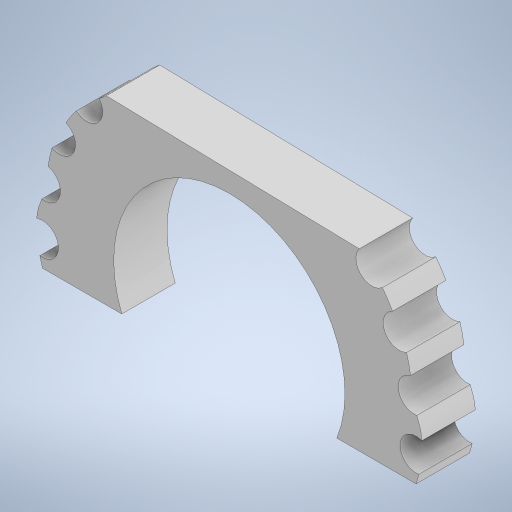
# Autodesk Inventor part: бок пуска держатель диодов
Saved by Autodesk Inventor 2023.1 (Build 271208000, 208)
## iProperties
Created: 2023-04-05
Part Number: бок пуска держатель диодов
Material: Типовые
Document SubType Name: Modeling
Designer: User
Density: 1 g/cm^3
Appearance: По умолчанию
Author: User
Autodesk Inventor part; units mm, degrees
(part 1 of 4)
ref_plane "YZ Plane" through (0, 0, 0) normal (1, 0, 0) x (0, 1, 0)
ref_plane "XZ Plane" through (0, 0, 0) normal (0, 1, 0) x (-1, 0, 0)
ref_plane "XY Plane" through (0, 0, 0) normal (0, 0, 1) x (1, 0, 0)
sketch "Эскиз1" plane through (0, 0, 0) normal (0, 0, 1) x (1, 0, 0)
  line L0 (-15.4323, 26.5556) -> (-15.4323, 37)
  line L1 (-15.4323, 37) -> (-36, 37)
  line L2 (-36, 37) -> (-36, 61)
  line L3 (-36, 61) -> (35, 61)
  line L4 (35, 61) -> (35, 37)
  line L5 (35, 37) -> (15.4323, 37)
  line L6 (15.4323, 37) -> (15.4323, 26.5556)
  line L7 (15.4323, 26.5556) -> (13.136, 23.9434)
  line L8 (11.832, 23.9746) -> (14.4323, 26.9326)
  line L9 (14.4323, 26.9326) -> (14.4323, 37)
  line L10 (14.4323, 37) -> (-14.4323, 37)
  line L11 (-14.4323, 37) -> (-14.4323, 26.9326)
  line L12 (-14.4323, 26.9326) -> (-12.3404, 24.5529)
  line L13 (-13.7005, 24.5855) -> (-15.4323, 26.5556)
  line L14 (39, 3.2152) -> (19.5419, 3.2152)
  line L15 (19.5419, 3.2152) -> (16.1608, 4.2152)
  line L16 (19.6867, 4.2152) -> (39, 4.2152)
  line L17 (39, 4.2152) -> (39, 63.4697)
  arc A0 (39, 63.4697) -> (38, 64.4697) centre (38, 63.4697) ccw
  line L18 (38, 64.4697) -> (10.2401, 64.4697)
  line L19 (10.2401, 64.4697) -> (10.2401, 65.4697)
  line L20 (10.2401, 65.4697) -> (38, 65.4697)
  arc A1 (40, 63.4697) -> (38, 65.4697) centre (38, 63.4697) ccw
  line L21 (40, 63.4697) -> (40, -99.0936)
  arc A2 (33, -106.0936) -> (40, -99.0936) centre (33, -99.0936) ccw
  line L22 (33, -106.0936) -> (-33, -106.0936)
  arc A3 (-40, -99.0936) -> (-33, -106.0936) centre (-33, -99.0936) ccw
  line L23 (-40, -99.0936) -> (-40, 63.4697)
  arc A4 (-38, 65.4697) -> (-40, 63.4697) centre (-38, 63.4697) ccw
  line L24 (-38, 65.4697) -> (-10.1221, 65.4697)
  line L25 (-10.1221, 65.4697) -> (-10.1221, 64.4697)
  line L26 (-10.1221, 64.4697) -> (-38, 64.4697)
  arc A5 (-38, 64.4697) -> (-39, 63.4697) centre (-38, 63.4697) ccw
  line L27 (-39, 63.4697) -> (-39, 4.2152)
  line L28 (-39, 4.2152) -> (-19.6867, 4.2152)
  line L29 (-16.1608, 4.2152) -> (-19.5419, 3.2152)
  line L30 (-19.5419, 3.2152) -> (-39, 3.2152)
  line L31 (-39, 3.2152) -> (-39, -99.0936)
  arc A6 (-39, -99.0936) -> (-33, -105.0936) centre (-33, -99.0936) ccw
  line L32 (-33, -105.0936) -> (33, -105.0936)
  arc A7 (33, -105.0936) -> (39, -99.0936) centre (33, -99.0936) ccw
  line L33 (39, -99.0936) -> (39, 3.2152)
  line L34 (34.3097, 25.5954) -> (34.3097, 24.7932)
  line L35 (34.3097, 24.7932) -> (34.257, 24.7932)
  line L36 (34.2611, 22.0622) -> (34.3097, 22.0622)
  line L37 (34.3097, 22.0622) -> (34.3097, 21.268)
  line L38 (27.8227, 25.9277) -> (28.6411, 25.9277)
  line L39 (28.6411, 25.9277) -> (30.3267, 20.9277)
  line L40 (30.3267, 20.9277) -> (29.6257, 20.9277)
  line L41 (29.6257, 20.9277) -> (29.1719, 22.3256)
  line L42 (29.1719, 22.3256) -> (27.2635, 22.3256)
  line L43 (27.2635, 22.3256) -> (26.8097, 20.9277)
  line L44 (26.8097, 20.9277) -> (26.1371, 20.9277)
  line L45 (26.1371, 20.9277) -> (27.8227, 25.9277)
  line L46 (24.0706, 20.9277) -> (22.6241, 20.9277)
  line L47 (22.6241, 20.9277) -> (22.6241, 25.9277)
  line L48 (22.6241, 25.9277) -> (25.6671, 25.9277)
  line L49 (25.6671, 25.9277) -> (25.6671, 25.3361)
  line L50 (25.6671, 25.3361) -> (23.2886, 25.3361)
  line L51 (23.2886, 25.3361) -> (23.2886, 23.9666)
  line L52 (23.2886, 23.9666) -> (24.0909, 23.9666)
  line L53 (26.6314, 29.3789) -> (26.6314, 30.0758)
  line L54 (26.6314, 30.0758) -> (26.6719, 30.0758)
  line L55 (27.8956, 30.8456) -> (27.4539, 30.8456)
  line L56 (27.4539, 30.8456) -> (27.4539, 31.3886)
  line L57 (27.4539, 31.3886) -> (27.7943, 31.3886)
  line L58 (26.8543, 32.1098) -> (26.8138, 32.1098)
  line L59 (26.8138, 32.1098) -> (26.8138, 32.7905)
  line L60 (24.7149, 32.9121) -> (26.0642, 32.9121)
  line L61 (26.0642, 32.9121) -> (26.0642, 29.1601)
  line L62 (26.0642, 29.1601) -> (25.4321, 29.1601)
  line L63 (25.4321, 29.1601) -> (25.4321, 30.6471)
  line L64 (25.4321, 30.6471) -> (24.8121, 30.6471)
  line L65 (24.8121, 30.6471) -> (23.6979, 29.1601)
  line L66 (23.6979, 29.1601) -> (22.9604, 29.1601)
  line L67 (22.9604, 29.1601) -> (24.1679, 30.7038)
  line L68 (19.1679, 32.7095) -> (19.1679, 32.0004)
  line L69 (19.1679, 32.0004) -> (19.1314, 32.0004)
  line L70 (19.1314, 30.0798) -> (19.1679, 30.0798)
  line L71 (19.1679, 30.0798) -> (19.1679, 29.3707)
  line L72 (-26.95, 20.6933) -> (-28.3965, 20.6933)
  line L73 (-28.3965, 20.6933) -> (-28.3965, 25.6933)
  line L74 (-28.3965, 25.6933) -> (-25.3535, 25.6933)
  line L75 (-25.3535, 25.6933) -> (-25.3535, 25.1017)
  line L76 (-25.3535, 25.1017) -> (-27.732, 25.1017)
  line L77 (-27.732, 25.1017) -> (-27.732, 23.7322)
  line L78 (-27.732, 23.7322) -> (-26.9297, 23.7322)
  line L79 (-37.0634, 29.1444) -> (-37.0634, 29.8414)
  line L80 (-37.0634, 29.8414) -> (-37.0229, 29.8414)
  line L81 (-35.7992, 30.6112) -> (-36.2409, 30.6112)
  line L82 (-36.2409, 30.6112) -> (-36.2409, 31.1542)
  line L83 (-36.2409, 31.1542) -> (-35.9005, 31.1542)
  line L84 (-36.8406, 31.8754) -> (-36.8811, 31.8754)
  line L85 (-36.8811, 31.8754) -> (-36.8811, 32.5561)
  line L86 (-33.4978, 31.9524) -> (-33.5342, 31.9524)
  line L87 (-33.5342, 31.9524) -> (-33.5342, 32.5966)
  line L88 (-30.8479, 31.4905) -> (-30.8479, 28.9256)
  line L89 (-30.8479, 28.9256) -> (-31.4799, 28.9256)
  line L90 (-31.4799, 28.9256) -> (-31.4799, 29.3227)
  line L91 (-29.3284, 29.1161) -> (-29.3284, 27.544)
  line L92 (-29.3284, 27.544) -> (-29.9605, 27.544)
  line L93 (-29.9605, 27.544) -> (-29.9605, 32.6777)
  line L94 (-29.9605, 32.6777) -> (-29.3284, 32.6777)
  line L95 (-29.3284, 32.6777) -> (-29.3284, 32.2846)
  line L96 (-24.7944, 32.6777) -> (-23.4451, 32.6777)
  line L97 (-23.4451, 32.6777) -> (-23.4451, 28.9256)
  line L98 (-23.4451, 28.9256) -> (-24.0772, 28.9256)
  line L99 (-24.0772, 28.9256) -> (-24.0772, 30.4127)
  line L100 (-24.0772, 30.4127) -> (-24.6971, 30.4127)
  line L101 (-24.6971, 30.4127) -> (-25.8114, 28.9256)
  line L102 (-25.8114, 28.9256) -> (-26.5488, 28.9256)
  line L103 (-26.5488, 28.9256) -> (-25.3414, 30.4694)
  line L104 (-21.9864, 32.6777) -> (-19.689, 32.6777)
  line L105 (-19.689, 32.6777) -> (-19.689, 29.4645)
  line L106 (-19.689, 29.4645) -> (-19.3162, 29.4645)
  line L107 (-19.3162, 29.4645) -> (-19.3162, 28.0261)
  line L108 (-19.3162, 28.0261) -> (-19.9038, 28.0261)
  line L109 (-19.9038, 28.0261) -> (-19.9038, 28.9337)
  line L110 (-19.9038, 28.9337) -> (-22.3714, 28.9337)
  line L111 (-22.3714, 28.9337) -> (-22.3714, 28.0261)
  line L112 (-22.3714, 28.0261) -> (-22.9589, 28.0261)
  line L113 (-22.9589, 28.0261) -> (-22.9589, 29.4645)
  line L114 (-22.9589, 29.4645) -> (-22.7117, 29.4645)
  line L115 (-35.5196, 25.6933) -> (-34.7012, 25.6933)
  line L116 (-34.7012, 25.6933) -> (-33.0156, 20.6933)
  line L117 (-33.0156, 20.6933) -> (-33.7166, 20.6933)
  line L118 (-33.7166, 20.6933) -> (-34.1704, 22.0912)
  line L119 (-34.1704, 22.0912) -> (-36.0788, 22.0912)
  line L120 (-36.0788, 22.0912) -> (-36.5326, 20.6933)
  line L121 (-36.5326, 20.6933) -> (-37.2052, 20.6933)
  line L122 (-37.2052, 20.6933) -> (-35.5196, 25.6933)
  line L123 (-30.8722, 23.3229) -> (-28.8422, 20.6933)
  line L124 (-28.8422, 20.6933) -> (-29.689, 20.6933)
  line L125 (-29.689, 20.6933) -> (-31.4597, 22.9866)
  line L126 (-31.4597, 22.9866) -> (-31.877, 22.9866)
  line L127 (-31.877, 22.9866) -> (-31.877, 20.6933)
  line L128 (-31.877, 20.6933) -> (-32.5415, 20.6933)
  line L129 (-32.5415, 20.6933) -> (-32.5415, 25.6933)
  line L130 (-32.5415, 25.6933) -> (-31.877, 25.6933)
  line L131 (-31.877, 25.6933) -> (-31.877, 23.4404)
  line L132 (-29.3122, 25.6933) -> (-29.1055, 25.6933)
  line L133 (-29.1055, 25.6933) -> (-29.1055, 25.1017)
  line L134 (-29.1055, 25.1017) -> (-29.2717, 25.1017)
  line L135 (21.2181, 29.1601) -> (19.7432, 29.1601)
  line L136 (19.7432, 29.1601) -> (19.7432, 32.9121)
  line L137 (19.7432, 32.9121) -> (21.1209, 32.9121)
  line L138 (31.4369, 29.1601) -> (30.1241, 29.1601)
  line L139 (30.1241, 29.1601) -> (30.1241, 32.9121)
  line L140 (30.1241, 32.9121) -> (30.7562, 32.9121)
  line L141 (30.7562, 32.9121) -> (30.7562, 31.4494)
  line L142 (30.7562, 31.4494) -> (31.4531, 31.4494)
  line L143 (38.3089, 32.7095) -> (38.3089, 32.0004)
  line L144 (38.3089, 32.0004) -> (38.2724, 32.0004)
  line L145 (38.2724, 30.0798) -> (38.3089, 30.0798)
  line L146 (38.3089, 30.0798) -> (38.3089, 29.3707)
  line L147 (36.0601, 21.9609) -> (36.1776, 22.2243)
  line L148 (36.1776, 22.2243) -> (34.4191, 25.9277)
  line L149 (34.4191, 25.9277) -> (35.1565, 25.9277)
  line L150 (35.1565, 25.9277) -> (36.5139, 22.986)
  line L151 (36.5139, 22.986) -> (37.7376, 25.9277)
  line L152 (37.7376, 25.9277) -> (38.4223, 25.9277)
  line L153 (38.4223, 25.9277) -> (36.6071, 21.7178)
  line L154 (34.9013, 20.9277) -> (34.9013, 21.5517)
  line L155 (34.9013, 21.5517) -> (34.9499, 21.5517)
  line L156 (-5.6509, -41.2421) -> (-5.6509, -36.154)
  line L157 (-5.6509, -36.154) -> (-8.0452, -36.154)
  line L158 (-8.0452, -36.154) -> (-8.0452, -41.2421)
  line L159 (-34.9687, -1.889) -> (-34.9687, -0.3964)
  line L160 (-34.9687, -0.3964) -> (-36.2158, -0.3964)
  line L161 (-36.2158, 0.1024) -> (-34.9687, 0.1024)
  line L162 (-34.9687, 0.1024) -> (-34.9687, 1.104)
  line L163 (-26.4317, -100.2362) -> (-26.4317, -101.232)
  line L164 (-26.4317, -101.232) -> (-26.032, -101.232)
  line L165 (-28.4267, -102.8274) -> (-29.2227, -102.8274)
  line L166 (-29.2227, -102.8274) -> (-29.2227, -103.8232)
  line L167 (5.095, 27.3433) -> (4.0974, 28.8866)
  line L168 (4.0974, 28.8866) -> (3.5401, 28.302)
  line L169 (3.5401, 28.302) -> (3.5401, 27.5031)
  line L170 (3.5401, 30.4961) -> (3.5401, 29.023)
  line L171 (3.5401, 29.023) -> (5.1223, 30.6831)
  line L172 (5.4497, 30.3051) -> (4.4481, 29.249)
  line L173 (4.4481, 29.249) -> (5.473, 27.6629)
  line L174 (-1.3976, 26.7549) -> (-1.3976, 27.2537)
  line L175 (-1.3976, 27.2537) -> (-2.3952, 27.2537)
  line L176 (-2.3952, 27.7525) -> (-1.3976, 27.7525)
  line L177 (-1.3976, 27.7525) -> (-1.3976, 30.4961)
  line L178 (6.3343, 34.5821) -> (6.3343, 33.335)
  line L179 (6.3343, 33.335) -> (7.8308, 33.335)
  line L180 (7.8308, 33.335) -> (7.8308, 34.5821)
  line L181 (7.8308, 31.5891) -> (7.8308, 32.8362)
  line L182 (7.8308, 32.8362) -> (6.3343, 32.8362)
  line L183 (6.3343, 32.8362) -> (6.3343, 31.5891)
  line L184 (4.5884, 32.8362) -> (2.8425, 32.8362)
  line L185 (2.8425, 32.8362) -> (2.8425, 32.3374)
  line L186 (-4.64, 31.5891) -> (-4.64, 34.3327)
  line L187 (-4.64, 34.3327) -> (-5.6376, 34.3327)
  line L188 (-5.6376, 34.3327) -> (-5.6376, 31.5891)
  line L189 (-3.6423, 34.3327) -> (-4.1411, 34.3327)
  line L190 (-4.1411, 34.3327) -> (-4.1411, 31.5891)
  line L191 (0.3136, 63.3342) -> (0.3136, 66.0778)
  line L192 (0.3136, 66.0778) -> (-0.2592, 66.0778)
  line L193 (-0.2592, 66.0778) -> (-1.1945, 63.2563)
  line L194 (-1.6778, 63.3225) -> (-1.6622, 63.4122)
  line L195 (-1.6622, 63.4122) -> (-0.6723, 66.4052)
  line L196 (-7.1688, 66.0778) -> (-8.1665, 66.0778)
  line L197 (-8.1665, 66.0778) -> (-8.1665, 63.3342)
  line L198 (4.0549, 64.5813) -> (2.309, 64.5813)
  line L199 (2.309, 64.5813) -> (2.309, 64.0825)
  line L200 (6.7984, 63.3342) -> (6.7984, 66.0778)
  line L201 (6.7984, 66.0778) -> (5.8008, 66.0778)
  line L202 (5.8008, 66.0778) -> (5.8008, 63.3342)
  line L203 (7.7961, 66.0778) -> (7.2973, 66.0778)
  line L204 (7.2973, 66.0778) -> (7.2973, 63.3342)
  line L205 (0.8472, 31.5891) -> (0.8472, 33.8066)
  line L206 (0.8472, 33.8066) -> (0.0521, 32.692)
  line L207 (-0.3532, 32.692) -> (-1.1482, 33.8066)
  line L208 (-1.1482, 33.8066) -> (-1.1482, 31.5891)
  line L209 (-1.1949, 34.7263) -> (-0.1505, 33.2649)
  line L210 (-0.1505, 33.2649) -> (0.8939, 34.7263)
  line L211 (-5.3882, 30.2467) -> (-6.3859, 30.2467)
  line L212 (-6.3859, 30.2467) -> (-6.3859, 27.5031)
  line L213 (-32.017, -102.6276) -> (-32.017, -100.436)
  line L214 (-32.017, -100.436) -> (-32.813, -100.436)
  line L215 (-32.813, -100.436) -> (-32.813, -102.6276)
  line L216 (-31.2177, -100.436) -> (-31.6174, -100.436)
  line L217 (-31.6174, -100.436) -> (-31.6174, -102.6276)
  line L218 (-23.9945, -2.6373) -> (-23.9945, 1.6028)
  line L219 (-23.9945, 1.6028) -> (-25.9898, 1.6028)
  line L220 (-25.9898, 1.6028) -> (-25.9898, -2.6373)
  line L221 (-0.8621, -40.3442) -> (-0.8621, -39.147)
  line L222 (-0.8621, -39.147) -> (-2.6579, -39.147)
  line L223 (-2.6579, -38.5484) -> (-0.8621, -38.5484)
  line L224 (-0.8621, -38.5484) -> (-0.8621, -35.8547)
  line L225 (5.7225, -35.8454) -> (5.7225, -38.1369)
  line L226 (5.7225, -38.1369) -> (8.2385, -35.6349)
  line L227 (8.6594, -36.0652) -> (6.8776, -37.8423)
  line L228 (6.8776, -37.8423) -> (8.7155, -41.0924)
  line L229 (8.7155, -41.0924) -> (8.7576, -41.2514)
  line L230 (8.187, -41.3824) -> (6.438, -38.2631)
  line L231 (6.438, -38.2631) -> (5.7225, -38.9646)
  line L232 (5.7225, -38.9646) -> (5.7225, -41.2421)
  line L233 (26.4641, 0.963) -> (26.659, 0.963)
  line L234 (26.659, 0.963) -> (25.5405, 2.027)
  line L235 (27.7112, 1.9607) -> (26.3394, 1.9607)
  line L236 (26.3394, 1.9607) -> (27.6605, 0.698)
  line L237 (27.6605, 0.698) -> (27.7229, 0.6162)
  line L238 (30.4548, -2.5288) -> (29.4571, -2.5288)
  line L239 (29.4571, -2.5288) -> (29.4571, -3.7758)
  arc A8 (-45, -109) -> (-42, -112) centre (-42, -109) ccw
  line L240 (-42, -112) -> (42, -112)
  arc A9 (42, -112) -> (45, -109) centre (42, -109) ccw
  line L241 (45, -109) -> (45, 108)
  arc A10 (45, 108) -> (42, 111) centre (42, 108) ccw
  line L242 (42, 111) -> (-42, 111)
  arc A11 (-42, 111) -> (-45, 108) centre (-42, 108) ccw
  line L243 (-45, 108) -> (-45, -109)
  line L244 (-30.3205, -53.3887) -> (-30.3205, -51.1972)
  line L245 (-30.3205, -51.1972) -> (-31.1165, -51.1972)
  line L246 (-31.1165, -51.1972) -> (-31.1165, -53.3887)
  line L247 (-29.5212, -51.1972) -> (-29.9208, -51.1972)
  line L248 (-29.9208, -51.1972) -> (-29.9208, -53.3887)
  arc A12 (37, 68) -> (40, 71) centre (37, 71) ccw
  line L249 (37, 68) -> (-37, 68)
  arc A13 (-40, 71) -> (-37, 68) centre (-37, 71) ccw
  line L250 (-40, 71) -> (-40, 102)
  arc A14 (-33, 109) -> (-40, 102) centre (-33, 102) ccw
  line L251 (-33, 109) -> (33, 109)
  arc A15 (40, 102) -> (33, 109) centre (33, 102) ccw
  line L252 (40, 102) -> (40, 71)
  circle A16 centre (-32, -94) radius 5
  circle A17 centre (-32, -44.7228) radius 5
  spline S0 degree 2 poles (31.1452, 21.4949) (30.8454, 21.8191) (30.5172, 22.7915) (30.5172, 23.4236) knots 0 0 0 1 2 2 2
  line L253 (31.1452, 21.4949) -> (30.8454, 21.8191) construction
  line L254 (30.8454, 21.8191) -> (30.5172, 22.7915) construction
  line L255 (30.5172, 22.7915) -> (30.5172, 23.4236) construction
  spline S1 degree 2 poles (30.5172, 23.4236) (30.5172, 24.0517) (30.8373, 24.9836) (31.1411, 25.328) knots 0 0 0 1 2 2 2
  line L256 (30.5172, 23.4236) -> (30.5172, 24.0517) construction
  line L257 (30.5172, 24.0517) -> (30.8373, 24.9836) construction
  line L258 (30.8373, 24.9836) -> (31.1411, 25.328) construction
  spline S2 degree 2 poles (31.1411, 25.328) (31.441, 25.6643) (32.2595, 26.0168) (32.7659, 26.0168) knots 0 0 0 1 2 2 2
  line L259 (31.1411, 25.328) -> (31.441, 25.6643) construction
  line L260 (31.441, 25.6643) -> (32.2595, 26.0168) construction
  line L261 (32.2595, 26.0168) -> (32.7659, 26.0168) construction
  spline S3 degree 2 poles (32.7659, 26.0168) (33.0172, 26.0168) (33.4588, 25.9439) (33.6452, 25.8872) knots 0 0 0 1 2 2 2
  line L262 (32.7659, 26.0168) -> (33.0172, 26.0168) construction
  line L263 (33.0172, 26.0168) -> (33.4588, 25.9439) construction
  line L264 (33.4588, 25.9439) -> (33.6452, 25.8872) construction
  spline S4 degree 2 poles (33.6452, 25.8872) (33.8073, 25.8345) (34.1436, 25.6846) (34.3097, 25.5954) knots 0 0 0 1 2 2 2
  line L265 (33.6452, 25.8872) -> (33.8073, 25.8345) construction
  line L266 (33.8073, 25.8345) -> (34.1436, 25.6846) construction
  line L267 (34.1436, 25.6846) -> (34.3097, 25.5954) construction
  spline S5 degree 2 poles (34.257, 24.7932) (34.1679, 24.8742) (33.8924, 25.1011) (33.6938, 25.2105) knots 0 0 0 1 2 2 2
  line L268 (34.257, 24.7932) -> (34.1679, 24.8742) construction
  line L269 (34.1679, 24.8742) -> (33.8924, 25.1011) construction
  line L270 (33.8924, 25.1011) -> (33.6938, 25.2105) construction
  spline S6 degree 2 poles (33.6938, 25.2105) (33.5034, 25.3159) (33.0536, 25.4496) (32.7619, 25.4496) knots 0 0 0 1 2 2 2
  line L271 (33.6938, 25.2105) -> (33.5034, 25.3159) construction
  line L272 (33.5034, 25.3159) -> (33.0536, 25.4496) construction
  line L273 (33.0536, 25.4496) -> (32.7619, 25.4496) construction
  spline S7 degree 2 poles (32.7619, 25.4496) (32.4418, 25.4496) (31.8705, 25.1862) (31.6557, 24.935) knots 0 0 0 1 2 2 2
  line L274 (32.7619, 25.4496) -> (32.4418, 25.4496) construction
  line L275 (32.4418, 25.4496) -> (31.8705, 25.1862) construction
  line L276 (31.8705, 25.1862) -> (31.6557, 24.935) construction
  spline S8 degree 2 poles (31.6557, 24.935) (31.445, 24.6797) (31.21, 23.9058) (31.21, 23.4236) knots 0 0 0 1 2 2 2
  line L277 (31.6557, 24.935) -> (31.445, 24.6797) construction
  line L278 (31.445, 24.6797) -> (31.21, 23.9058) construction
  line L279 (31.21, 23.9058) -> (31.21, 23.4236) construction
  spline S9 degree 2 poles (31.21, 23.4236) (31.21, 22.909) (31.4572, 22.1676) (31.6719, 21.9123) knots 0 0 0 1 2 2 2
  line L280 (31.21, 23.4236) -> (31.21, 22.909) construction
  line L281 (31.21, 22.909) -> (31.4572, 22.1676) construction
  line L282 (31.4572, 22.1676) -> (31.6719, 21.9123) construction
  spline S10 degree 2 poles (31.6719, 21.9123) (31.8826, 21.6651) (32.4458, 21.4139) (32.7619, 21.4139) knots 0 0 0 1 2 2 2
  line L283 (31.6719, 21.9123) -> (31.8826, 21.6651) construction
  line L284 (31.8826, 21.6651) -> (32.4458, 21.4139) construction
  line L285 (32.4458, 21.4139) -> (32.7619, 21.4139) construction
  spline S11 degree 2 poles (32.7619, 21.4139) (33.0496, 21.4139) (33.5398, 21.5557) (33.7303, 21.6611) knots 0 0 0 1 2 2 2
  line L286 (32.7619, 21.4139) -> (33.0496, 21.4139) construction
  line L287 (33.0496, 21.4139) -> (33.5398, 21.5557) construction
  line L288 (33.5398, 21.5557) -> (33.7303, 21.6611) construction
  spline S12 degree 2 poles (33.7303, 21.6611) (33.9126, 21.7664) (34.1841, 21.9852) (34.2611, 22.0622) knots 0 0 0 1 2 2 2
  line L289 (33.7303, 21.6611) -> (33.9126, 21.7664) construction
  line L290 (33.9126, 21.7664) -> (34.1841, 21.9852) construction
  line L291 (34.1841, 21.9852) -> (34.2611, 22.0622) construction
  spline S13 degree 2 poles (34.3097, 21.268) (34.1436, 21.1911) (33.8518, 21.0492) (33.6452, 20.9844) knots 0 0 0 1 2 2 2
  line L292 (34.3097, 21.268) -> (34.1436, 21.1911) construction
  line L293 (34.1436, 21.1911) -> (33.8518, 21.0492) construction
  line L294 (33.8518, 21.0492) -> (33.6452, 20.9844) construction
  spline S14 degree 2 poles (33.6452, 20.9844) (33.4264, 20.9115) (33.0536, 20.8385) (32.7538, 20.8385) knots 0 0 0 1 2 2 2
  line L295 (33.6452, 20.9844) -> (33.4264, 20.9115) construction
  line L296 (33.4264, 20.9115) -> (33.0536, 20.8385) construction
  line L297 (33.0536, 20.8385) -> (32.7538, 20.8385) construction
  spline S15 degree 2 poles (32.7538, 20.8385) (32.2676, 20.8385) (31.445, 21.1667) (31.1452, 21.4949) knots 0 0 0 1 2 2 2
  line L298 (32.7538, 20.8385) -> (32.2676, 20.8385) construction
  line L299 (32.2676, 20.8385) -> (31.445, 21.1667) construction
  line L300 (31.445, 21.1667) -> (31.1452, 21.4949) construction
  spline S16 degree 2 poles (25.509, 21.3369) (25.2254, 21.1141) (24.5812, 20.9277) (24.0706, 20.9277) knots 0 0 0 1 2 2 2
  line L301 (25.509, 21.3369) -> (25.2254, 21.1141) construction
  line L302 (25.2254, 21.1141) -> (24.5812, 20.9277) construction
  line L303 (24.5812, 20.9277) -> (24.0706, 20.9277) construction
  spline S17 degree 2 poles (24.0909, 23.9666) (24.6014, 23.9666) (25.2457, 23.8491) (25.5293, 23.6262) knots 0 0 0 1 2 2 2
  line L304 (24.0909, 23.9666) -> (24.6014, 23.9666) construction
  line L305 (24.6014, 23.9666) -> (25.2457, 23.8491) construction
  line L306 (25.2457, 23.8491) -> (25.5293, 23.6262) construction
  spline S18 degree 2 poles (25.5293, 23.6262) (25.7846, 23.4277) (26.0277, 22.8442) (26.0277, 22.4755) knots 0 0 0 1 2 2 2
  line L307 (25.5293, 23.6262) -> (25.7846, 23.4277) construction
  line L308 (25.7846, 23.4277) -> (26.0277, 22.8442) construction
  line L309 (26.0277, 22.8442) -> (26.0277, 22.4755) construction
  spline S19 degree 2 poles (26.0277, 22.4755) (26.0277, 22.1149) (25.7441, 21.5233) (25.509, 21.3369) knots 0 0 0 1 2 2 2
  line L310 (26.0277, 22.4755) -> (26.0277, 22.1149) construction
  line L311 (26.0277, 22.1149) -> (25.7441, 21.5233) construction
  line L312 (25.7441, 21.5233) -> (25.509, 21.3369) construction
  spline S20 degree 2 poles (28.9693, 29.3221) (28.7667, 29.1965) (28.2441, 29.075) (27.9807, 29.075) knots 0 0 0 1 2 2 2
  line L313 (28.9693, 29.3221) -> (28.7667, 29.1965) construction
  line L314 (28.7667, 29.1965) -> (28.2441, 29.075) construction
  line L315 (28.2441, 29.075) -> (27.9807, 29.075) construction
  spline S21 degree 2 poles (27.9807, 29.075) (27.612, 29.075) (26.9556, 29.2208) (26.6314, 29.3789) knots 0 0 0 1 2 2 2
  line L316 (27.9807, 29.075) -> (27.612, 29.075) construction
  line L317 (27.612, 29.075) -> (26.9556, 29.2208) construction
  line L318 (26.9556, 29.2208) -> (26.6314, 29.3789) construction
  spline S22 degree 2 poles (26.6719, 30.0758) (26.8988, 29.8651) (27.5877, 29.6179) (27.928, 29.6179) knots 0 0 0 1 2 2 2
  line L319 (26.6719, 30.0758) -> (26.8988, 29.8651) construction
  line L320 (26.8988, 29.8651) -> (27.5877, 29.6179) construction
  line L321 (27.5877, 29.6179) -> (27.928, 29.6179) construction
  spline S23 degree 2 poles (27.928, 29.6179) (28.0739, 29.6179) (28.4142, 29.6827) (28.5317, 29.7476) knots 0 0 0 1 2 2 2
  line L322 (27.928, 29.6179) -> (28.0739, 29.6179) construction
  line L323 (28.0739, 29.6179) -> (28.4142, 29.6827) construction
  line L324 (28.4142, 29.6827) -> (28.5317, 29.7476) construction
  spline S24 degree 2 poles (28.5317, 29.7476) (28.6857, 29.8448) (28.8154, 30.0596) (28.8154, 30.246) knots 0 0 0 1 2 2 2
  line L325 (28.5317, 29.7476) -> (28.6857, 29.8448) construction
  line L326 (28.6857, 29.8448) -> (28.8154, 30.0596) construction
  line L327 (28.8154, 30.0596) -> (28.8154, 30.246) construction
  spline S25 degree 2 poles (28.8154, 30.246) (28.8154, 30.4485) (28.6655, 30.6957) (28.5317, 30.7565) knots 0 0 0 1 2 2 2
  line L328 (28.8154, 30.246) -> (28.8154, 30.4485) construction
  line L329 (28.8154, 30.4485) -> (28.6655, 30.6957) construction
  line L330 (28.6655, 30.6957) -> (28.5317, 30.7565) construction
  spline S26 degree 2 poles (28.5317, 30.7565) (28.4021, 30.8173) (28.0779, 30.8456) (27.8956, 30.8456) knots 0 0 0 1 2 2 2
  line L331 (28.5317, 30.7565) -> (28.4021, 30.8173) construction
  line L332 (28.4021, 30.8173) -> (28.0779, 30.8456) construction
  line L333 (28.0779, 30.8456) -> (27.8956, 30.8456) construction
  spline S27 degree 2 poles (27.7943, 31.3886) (27.9199, 31.3886) (28.3008, 31.4048) (28.4142, 31.4494) knots 0 0 0 1 2 2 2
  line L334 (27.7943, 31.3886) -> (27.9199, 31.3886) construction
  line L335 (27.9199, 31.3886) -> (28.3008, 31.4048) construction
  line L336 (28.3008, 31.4048) -> (28.4142, 31.4494) construction
  spline S28 degree 2 poles (28.4142, 31.4494) (28.5601, 31.502) (28.7343, 31.7006) (28.7343, 31.9356) knots 0 0 0 1 2 2 2
  line L337 (28.4142, 31.4494) -> (28.5601, 31.502) construction
  line L338 (28.5601, 31.502) -> (28.7343, 31.7006) construction
  line L339 (28.7343, 31.7006) -> (28.7343, 31.9356) construction
  spline S29 degree 2 poles (28.7343, 31.9356) (28.7343, 32.1017) (28.5885, 32.3002) (28.475, 32.357) knots 0 0 0 1 2 2 2
  line L340 (28.7343, 31.9356) -> (28.7343, 32.1017) construction
  line L341 (28.7343, 32.1017) -> (28.5885, 32.3002) construction
  line L342 (28.5885, 32.3002) -> (28.475, 32.357) construction
  spline S30 degree 2 poles (28.475, 32.357) (28.3616, 32.4177) (28.0941, 32.4623) (27.9685, 32.4623) knots 0 0 0 1 2 2 2
  line L343 (28.475, 32.357) -> (28.3616, 32.4177) construction
  line L344 (28.3616, 32.4177) -> (28.0941, 32.4623) construction
  line L345 (28.0941, 32.4623) -> (27.9685, 32.4623) construction
  spline S31 degree 2 poles (27.9685, 32.4623) (27.6525, 32.4623) (27.065, 32.284) (26.8543, 32.1098) knots 0 0 0 1 2 2 2
  line L346 (27.9685, 32.4623) -> (27.6525, 32.4623) construction
  line L347 (27.6525, 32.4623) -> (27.065, 32.284) construction
  line L348 (27.065, 32.284) -> (26.8543, 32.1098) construction
  spline S32 degree 2 poles (26.8138, 32.7905) (27.0569, 32.8756) (27.6403, 33.0012) (27.9361, 33.0012) knots 0 0 0 1 2 2 2
  line L349 (26.8138, 32.7905) -> (27.0569, 32.8756) construction
  line L350 (27.0569, 32.8756) -> (27.6403, 33.0012) construction
  line L351 (27.6403, 33.0012) -> (27.9361, 33.0012) construction
  spline S33 degree 2 poles (27.9361, 33.0012) (28.1752, 33.0012) (28.6695, 32.904) (28.8883, 32.7865) knots 0 0 0 1 2 2 2
  line L352 (27.9361, 33.0012) -> (28.1752, 33.0012) construction
  line L353 (28.1752, 33.0012) -> (28.6695, 32.904) construction
  line L354 (28.6695, 32.904) -> (28.8883, 32.7865) construction
  spline S34 degree 2 poles (28.8883, 32.7865) (29.099, 32.673) (29.3786, 32.2719) (29.3786, 31.9842) knots 0 0 0 1 2 2 2
  line L355 (28.8883, 32.7865) -> (29.099, 32.673) construction
  line L356 (29.099, 32.673) -> (29.3786, 32.2719) construction
  line L357 (29.3786, 32.2719) -> (29.3786, 31.9842) construction
  spline S35 degree 2 poles (29.3786, 31.9842) (29.3786, 31.6803) (29.0342, 31.2224) (28.7505, 31.1455) knots 0 0 0 1 2 2 2
  line L358 (29.3786, 31.9842) -> (29.3786, 31.6803) construction
  line L359 (29.3786, 31.6803) -> (29.0342, 31.2224) construction
  line L360 (29.0342, 31.2224) -> (28.7505, 31.1455) construction
  line L361 (28.7505, 31.1455) -> (28.7505, 31.1252)
  spline S36 degree 2 poles (28.7505, 31.1252) (29.0625, 31.0158) (29.4596, 30.5742) (29.4596, 30.2014) knots 0 0 0 1 2 2 2
  line L362 (28.7505, 31.1252) -> (29.0625, 31.0158) construction
  line L363 (29.0625, 31.0158) -> (29.4596, 30.5742) construction
  line L364 (29.4596, 30.5742) -> (29.4596, 30.2014) construction
  spline S37 degree 2 poles (29.4596, 30.2014) (29.4596, 29.8853) (29.1841, 29.4477) (28.9693, 29.3221) knots 0 0 0 1 2 2 2
  line L365 (29.4596, 30.2014) -> (29.4596, 29.8853) construction
  line L366 (29.4596, 29.8853) -> (29.1841, 29.4477) construction
  line L367 (29.1841, 29.4477) -> (28.9693, 29.3221) construction
  spline S38 degree 2 poles (24.1679, 30.7038) (23.6979, 30.8416) (23.2643, 31.3845) (23.2643, 31.8424) knots 0 0 0 1 2 2 2
  line L368 (24.1679, 30.7038) -> (23.6979, 30.8416) construction
  line L369 (23.6979, 30.8416) -> (23.2643, 31.3845) construction
  line L370 (23.2643, 31.3845) -> (23.2643, 31.8424) construction
  spline S39 degree 2 poles (23.2643, 31.8424) (23.2643, 32.122) (23.5115, 32.5434) (23.7181, 32.6852) knots 0 0 0 1 2 2 2
  line L371 (23.2643, 31.8424) -> (23.2643, 32.122) construction
  line L372 (23.2643, 32.122) -> (23.5115, 32.5434) construction
  line L373 (23.5115, 32.5434) -> (23.7181, 32.6852) construction
  spline S40 degree 2 poles (23.7181, 32.6852) (23.8843, 32.8027) (24.3988, 32.9121) (24.7149, 32.9121) knots 0 0 0 1 2 2 2
  line L374 (23.7181, 32.6852) -> (23.8843, 32.8027) construction
  line L375 (23.8843, 32.8027) -> (24.3988, 32.9121) construction
  line L376 (24.3988, 32.9121) -> (24.7149, 32.9121) construction
  spline S41 degree 2 poles (16.7975, 29.5571) (16.5666, 29.7962) (16.3113, 30.5336) (16.3113, 31.028) knots 0 0 0 1 2 2 2
  line L377 (16.7975, 29.5571) -> (16.5666, 29.7962) construction
  line L378 (16.5666, 29.7962) -> (16.3113, 30.5336) construction
  line L379 (16.3113, 30.5336) -> (16.3113, 31.028) construction
  spline S42 degree 2 poles (16.3113, 31.028) (16.3113, 31.5223) (16.5747, 32.2435) (16.7975, 32.4866) knots 0 0 0 1 2 2 2
  line L380 (16.3113, 31.028) -> (16.3113, 31.5223) construction
  line L381 (16.3113, 31.5223) -> (16.5747, 32.2435) construction
  line L382 (16.5747, 32.2435) -> (16.7975, 32.4866) construction
  spline S43 degree 2 poles (16.7975, 32.4866) (17.0204, 32.7338) (17.6808, 32.9972) (18.0617, 32.9972) knots 0 0 0 1 2 2 2
  line L383 (16.7975, 32.4866) -> (17.0204, 32.7338) construction
  line L384 (17.0204, 32.7338) -> (17.6808, 32.9972) construction
  line L385 (17.6808, 32.9972) -> (18.0617, 32.9972) construction
  spline S44 degree 2 poles (18.0617, 32.9972) (18.3697, 32.9972) (18.945, 32.8229) (19.1679, 32.7095) knots 0 0 0 1 2 2 2
  line L386 (18.0617, 32.9972) -> (18.3697, 32.9972) construction
  line L387 (18.3697, 32.9972) -> (18.945, 32.8229) construction
  line L388 (18.945, 32.8229) -> (19.1679, 32.7095) construction
  spline S45 degree 2 poles (19.1314, 32.0004) (19.0625, 32.0571) (18.8518, 32.203) (18.7019, 32.28) knots 0 0 0 1 2 2 2
  line L389 (19.1314, 32.0004) -> (19.0625, 32.0571) construction
  line L390 (19.0625, 32.0571) -> (18.8518, 32.203) construction
  line L391 (18.8518, 32.203) -> (18.7019, 32.28) construction
  spline S46 degree 2 poles (18.7019, 32.28) (18.5682, 32.3448) (18.2116, 32.4461) (18.0496, 32.4461) knots 0 0 0 1 2 2 2
  line L392 (18.7019, 32.28) -> (18.5682, 32.3448) construction
  line L393 (18.5682, 32.3448) -> (18.2116, 32.4461) construction
  line L394 (18.2116, 32.4461) -> (18.0496, 32.4461) construction
  spline S47 degree 2 poles (18.0496, 32.4461) (17.5593, 32.4461) (16.9637, 31.7046) (16.9637, 31.028) knots 0 0 0 1 2 2 2
  line L395 (18.0496, 32.4461) -> (17.5593, 32.4461) construction
  line L396 (17.5593, 32.4461) -> (16.9637, 31.7046) construction
  line L397 (16.9637, 31.7046) -> (16.9637, 31.028) construction
  spline S48 degree 2 poles (16.9637, 31.028) (16.9637, 30.3675) (17.539, 29.626) (18.0496, 29.626) knots 0 0 0 1 2 2 2
  line L398 (16.9637, 31.028) -> (16.9637, 30.3675) construction
  line L399 (16.9637, 30.3675) -> (17.539, 29.626) construction
  line L400 (17.539, 29.626) -> (18.0496, 29.626) construction
  spline S49 degree 2 poles (18.0496, 29.626) (18.3575, 29.626) (18.9167, 29.8813) (19.1314, 30.0798) knots 0 0 0 1 2 2 2
  line L401 (18.0496, 29.626) -> (18.3575, 29.626) construction
  line L402 (18.3575, 29.626) -> (18.9167, 29.8813) construction
  line L403 (18.9167, 29.8813) -> (19.1314, 30.0798) construction
  spline S50 degree 2 poles (19.1679, 29.3707) (19.0747, 29.3262) (18.7911, 29.2006) (18.6776, 29.1722) knots 0 0 0 1 2 2 2
  line L404 (19.1679, 29.3707) -> (19.0747, 29.3262) construction
  line L405 (19.0747, 29.3262) -> (18.7911, 29.2006) construction
  line L406 (18.7911, 29.2006) -> (18.6776, 29.1722) construction
  spline S51 degree 2 poles (18.6776, 29.1722) (18.5155, 29.1236) (18.2603, 29.075) (18.0617, 29.075) knots 0 0 0 1 2 2 2
  line L407 (18.6776, 29.1722) -> (18.5155, 29.1236) construction
  line L408 (18.5155, 29.1236) -> (18.2603, 29.075) construction
  line L409 (18.2603, 29.075) -> (18.0617, 29.075) construction
  spline S52 degree 2 poles (18.0617, 29.075) (17.6727, 29.075) (17.0285, 29.314) (16.7975, 29.5571) knots 0 0 0 1 2 2 2
  line L410 (18.0617, 29.075) -> (17.6727, 29.075) construction
  line L411 (17.6727, 29.075) -> (17.0285, 29.314) construction
  line L412 (17.0285, 29.314) -> (16.7975, 29.5571) construction
  spline S53 degree 2 poles (-25.5115, 21.1025) (-25.7952, 20.8797) (-26.4394, 20.6933) (-26.95, 20.6933) knots 0 0 0 1 2 2 2
  line L413 (-25.5115, 21.1025) -> (-25.7952, 20.8797) construction
  line L414 (-25.7952, 20.8797) -> (-26.4394, 20.6933) construction
  line L415 (-26.4394, 20.6933) -> (-26.95, 20.6933) construction
  spline S54 degree 2 poles (-26.9297, 23.7322) (-26.4192, 23.7322) (-25.7749, 23.6147) (-25.4913, 23.3918) knots 0 0 0 1 2 2 2
  line L416 (-26.9297, 23.7322) -> (-26.4192, 23.7322) construction
  line L417 (-26.4192, 23.7322) -> (-25.7749, 23.6147) construction
  line L418 (-25.7749, 23.6147) -> (-25.4913, 23.3918) construction
  spline S55 degree 2 poles (-25.4913, 23.3918) (-25.236, 23.1933) (-24.9929, 22.6098) (-24.9929, 22.2411) knots 0 0 0 1 2 2 2
  line L419 (-25.4913, 23.3918) -> (-25.236, 23.1933) construction
  line L420 (-25.236, 23.1933) -> (-24.9929, 22.6098) construction
  line L421 (-24.9929, 22.6098) -> (-24.9929, 22.2411) construction
  spline S56 degree 2 poles (-24.9929, 22.2411) (-24.9929, 21.8805) (-25.2765, 21.2889) (-25.5115, 21.1025) knots 0 0 0 1 2 2 2
  line L422 (-24.9929, 22.2411) -> (-24.9929, 21.8805) construction
  line L423 (-24.9929, 21.8805) -> (-25.2765, 21.2889) construction
  line L424 (-25.2765, 21.2889) -> (-25.5115, 21.1025) construction
  spline S57 degree 2 poles (-34.7255, 29.0877) (-34.9281, 28.9621) (-35.4508, 28.8406) (-35.7141, 28.8406) knots 0 0 0 1 2 2 2
  line L425 (-34.7255, 29.0877) -> (-34.9281, 28.9621) construction
  line L426 (-34.9281, 28.9621) -> (-35.4508, 28.8406) construction
  line L427 (-35.4508, 28.8406) -> (-35.7141, 28.8406) construction
  spline S58 degree 2 poles (-35.7141, 28.8406) (-36.0829, 28.8406) (-36.7393, 28.9864) (-37.0634, 29.1444) knots 0 0 0 1 2 2 2
  line L428 (-35.7141, 28.8406) -> (-36.0829, 28.8406) construction
  line L429 (-36.0829, 28.8406) -> (-36.7393, 28.9864) construction
  line L430 (-36.7393, 28.9864) -> (-37.0634, 29.1444) construction
  spline S59 degree 2 poles (-37.0229, 29.8414) (-36.796, 29.6307) (-36.1072, 29.3835) (-35.7668, 29.3835) knots 0 0 0 1 2 2 2
  line L431 (-37.0229, 29.8414) -> (-36.796, 29.6307) construction
  line L432 (-36.796, 29.6307) -> (-36.1072, 29.3835) construction
  line L433 (-36.1072, 29.3835) -> (-35.7668, 29.3835) construction
  spline S60 degree 2 poles (-35.7668, 29.3835) (-35.6209, 29.3835) (-35.2806, 29.4483) (-35.1631, 29.5132) knots 0 0 0 1 2 2 2
  line L434 (-35.7668, 29.3835) -> (-35.6209, 29.3835) construction
  line L435 (-35.6209, 29.3835) -> (-35.2806, 29.4483) construction
  line L436 (-35.2806, 29.4483) -> (-35.1631, 29.5132) construction
  spline S61 degree 2 poles (-35.1631, 29.5132) (-35.0091, 29.6104) (-34.8795, 29.8252) (-34.8795, 30.0115) knots 0 0 0 1 2 2 2
  line L437 (-35.1631, 29.5132) -> (-35.0091, 29.6104) construction
  line L438 (-35.0091, 29.6104) -> (-34.8795, 29.8252) construction
  line L439 (-34.8795, 29.8252) -> (-34.8795, 30.0115) construction
  spline S62 degree 2 poles (-34.8795, 30.0115) (-34.8795, 30.2141) (-35.0294, 30.4613) (-35.1631, 30.5221) knots 0 0 0 1 2 2 2
  line L440 (-34.8795, 30.0115) -> (-34.8795, 30.2141) construction
  line L441 (-34.8795, 30.2141) -> (-35.0294, 30.4613) construction
  line L442 (-35.0294, 30.4613) -> (-35.1631, 30.5221) construction
  spline S63 degree 2 poles (-35.1631, 30.5221) (-35.2927, 30.5829) (-35.6169, 30.6112) (-35.7992, 30.6112) knots 0 0 0 1 2 2 2
  line L443 (-35.1631, 30.5221) -> (-35.2927, 30.5829) construction
  line L444 (-35.2927, 30.5829) -> (-35.6169, 30.6112) construction
  line L445 (-35.6169, 30.6112) -> (-35.7992, 30.6112) construction
  spline S64 degree 2 poles (-35.9005, 31.1542) (-35.7749, 31.1542) (-35.394, 31.1704) (-35.2806, 31.2149) knots 0 0 0 1 2 2 2
  line L446 (-35.9005, 31.1542) -> (-35.7749, 31.1542) construction
  line L447 (-35.7749, 31.1542) -> (-35.394, 31.1704) construction
  line L448 (-35.394, 31.1704) -> (-35.2806, 31.2149) construction
  spline S65 degree 2 poles (-35.2806, 31.2149) (-35.1347, 31.2676) (-34.9605, 31.4662) (-34.9605, 31.7012) knots 0 0 0 1 2 2 2
  line L449 (-35.2806, 31.2149) -> (-35.1347, 31.2676) construction
  line L450 (-35.1347, 31.2676) -> (-34.9605, 31.4662) construction
  line L451 (-34.9605, 31.4662) -> (-34.9605, 31.7012) construction
  spline S66 degree 2 poles (-34.9605, 31.7012) (-34.9605, 31.8673) (-35.1064, 32.0658) (-35.2198, 32.1226) knots 0 0 0 1 2 2 2
  line L452 (-34.9605, 31.7012) -> (-34.9605, 31.8673) construction
  line L453 (-34.9605, 31.8673) -> (-35.1064, 32.0658) construction
  line L454 (-35.1064, 32.0658) -> (-35.2198, 32.1226) construction
  spline S67 degree 2 poles (-35.2198, 32.1226) (-35.3333, 32.1833) (-35.6007, 32.2279) (-35.7263, 32.2279) knots 0 0 0 1 2 2 2
  line L455 (-35.2198, 32.1226) -> (-35.3333, 32.1833) construction
  line L456 (-35.3333, 32.1833) -> (-35.6007, 32.2279) construction
  line L457 (-35.6007, 32.2279) -> (-35.7263, 32.2279) construction
  spline S68 degree 2 poles (-35.7263, 32.2279) (-36.0423, 32.2279) (-36.6299, 32.0496) (-36.8406, 31.8754) knots 0 0 0 1 2 2 2
  line L458 (-35.7263, 32.2279) -> (-36.0423, 32.2279) construction
  line L459 (-36.0423, 32.2279) -> (-36.6299, 32.0496) construction
  line L460 (-36.6299, 32.0496) -> (-36.8406, 31.8754) construction
  spline S69 degree 2 poles (-36.8811, 32.5561) (-36.638, 32.6412) (-36.0545, 32.7668) (-35.7587, 32.7668) knots 0 0 0 1 2 2 2
  line L461 (-36.8811, 32.5561) -> (-36.638, 32.6412) construction
  line L462 (-36.638, 32.6412) -> (-36.0545, 32.7668) construction
  line L463 (-36.0545, 32.7668) -> (-35.7587, 32.7668) construction
  spline S70 degree 2 poles (-35.7587, 32.7668) (-35.5196, 32.7668) (-35.0253, 32.6696) (-34.8065, 32.5521) knots 0 0 0 1 2 2 2
  line L464 (-35.7587, 32.7668) -> (-35.5196, 32.7668) construction
  line L465 (-35.5196, 32.7668) -> (-35.0253, 32.6696) construction
  line L466 (-35.0253, 32.6696) -> (-34.8065, 32.5521) construction
  spline S71 degree 2 poles (-34.8065, 32.5521) (-34.5958, 32.4386) (-34.3162, 32.0375) (-34.3162, 31.7498) knots 0 0 0 1 2 2 2
  line L467 (-34.8065, 32.5521) -> (-34.5958, 32.4386) construction
  line L468 (-34.5958, 32.4386) -> (-34.3162, 32.0375) construction
  line L469 (-34.3162, 32.0375) -> (-34.3162, 31.7498) construction
  spline S72 degree 2 poles (-34.3162, 31.7498) (-34.3162, 31.4459) (-34.6607, 30.988) (-34.9443, 30.9111) knots 0 0 0 1 2 2 2
  line L470 (-34.3162, 31.7498) -> (-34.3162, 31.4459) construction
  line L471 (-34.3162, 31.4459) -> (-34.6607, 30.988) construction
  line L472 (-34.6607, 30.988) -> (-34.9443, 30.9111) construction
  line L473 (-34.9443, 30.9111) -> (-34.9443, 30.8908)
  spline S73 degree 2 poles (-34.9443, 30.8908) (-34.6323, 30.7814) (-34.2352, 30.3397) (-34.2352, 29.967) knots 0 0 0 1 2 2 2
  line L474 (-34.9443, 30.8908) -> (-34.6323, 30.7814) construction
  line L475 (-34.6323, 30.7814) -> (-34.2352, 30.3397) construction
  line L476 (-34.2352, 30.3397) -> (-34.2352, 29.967) construction
  spline S74 degree 2 poles (-34.2352, 29.967) (-34.2352, 29.6509) (-34.5107, 29.2133) (-34.7255, 29.0877) knots 0 0 0 1 2 2 2
  line L477 (-34.2352, 29.967) -> (-34.2352, 29.6509) construction
  line L478 (-34.2352, 29.6509) -> (-34.5107, 29.2133) construction
  line L479 (-34.5107, 29.2133) -> (-34.7255, 29.0877) construction
  spline S75 degree 2 poles (-31.9378, 29.0026) (-32.1039, 28.9135) (-32.4159, 28.8203) (-32.6996, 28.8203) knots 0 0 0 1 2 2 2
  line L480 (-31.9378, 29.0026) -> (-32.1039, 28.9135) construction
  line L481 (-32.1039, 28.9135) -> (-32.4159, 28.8203) construction
  line L482 (-32.4159, 28.8203) -> (-32.6996, 28.8203) construction
  spline S76 degree 2 poles (-32.6996, 28.8203) (-32.9305, 28.8203) (-33.3479, 28.9945) (-33.5059, 29.1525) knots 0 0 0 1 2 2 2
  line L483 (-32.6996, 28.8203) -> (-32.9305, 28.8203) construction
  line L484 (-32.9305, 28.8203) -> (-33.3479, 28.9945) construction
  line L485 (-33.3479, 28.9945) -> (-33.5059, 29.1525) construction
  spline S77 degree 2 poles (-33.5059, 29.1525) (-33.6558, 29.3065) (-33.8381, 29.7603) (-33.8381, 30.0115) knots 0 0 0 1 2 2 2
  line L486 (-33.5059, 29.1525) -> (-33.6558, 29.3065) construction
  line L487 (-33.6558, 29.3065) -> (-33.8381, 29.7603) construction
  line L488 (-33.8381, 29.7603) -> (-33.8381, 30.0115) construction
  spline S78 degree 2 poles (-33.8381, 30.0115) (-33.8381, 30.4005) (-33.5099, 30.9516) (-33.1534, 31.1096) knots 0 0 0 1 2 2 2
  line L489 (-33.8381, 30.0115) -> (-33.8381, 30.4005) construction
  line L490 (-33.8381, 30.4005) -> (-33.5099, 30.9516) construction
  line L491 (-33.5099, 30.9516) -> (-33.1534, 31.1096) construction
  spline S79 degree 2 poles (-33.1534, 31.1096) (-32.8373, 31.2555) (-31.9783, 31.3649) (-31.4799, 31.3932) knots 0 0 0 1 2 2 2
  line L492 (-33.1534, 31.1096) -> (-32.8373, 31.2555) construction
  line L493 (-32.8373, 31.2555) -> (-31.9783, 31.3649) construction
  line L494 (-31.9783, 31.3649) -> (-31.4799, 31.3932) construction
  line L495 (-31.4799, 31.3932) -> (-31.4799, 31.5148)
  spline S80 degree 2 poles (-31.4799, 31.5148) (-31.4799, 31.7336) (-31.6137, 32.0051) (-31.7352, 32.082) knots 0 0 0 1 2 2 2
  line L496 (-31.4799, 31.5148) -> (-31.4799, 31.7336) construction
  line L497 (-31.4799, 31.7336) -> (-31.6137, 32.0051) construction
  line L498 (-31.6137, 32.0051) -> (-31.7352, 32.082) construction
  spline S81 degree 2 poles (-31.7352, 32.082) (-31.8568, 32.159) (-32.2052, 32.2077) (-32.3916, 32.2077) knots 0 0 0 1 2 2 2
  line L499 (-31.7352, 32.082) -> (-31.8568, 32.159) construction
  line L500 (-31.8568, 32.159) -> (-32.2052, 32.2077) construction
  line L501 (-32.2052, 32.2077) -> (-32.3916, 32.2077) construction
  spline S82 degree 2 poles (-32.3916, 32.2077) (-32.6104, 32.2077) (-33.202, 32.078) (-33.4978, 31.9524) knots 0 0 0 1 2 2 2
  line L502 (-32.3916, 32.2077) -> (-32.6104, 32.2077) construction
  line L503 (-32.6104, 32.2077) -> (-33.202, 32.078) construction
  line L504 (-33.202, 32.078) -> (-33.4978, 31.9524) construction
  spline S83 degree 2 poles (-33.5342, 32.5966) (-33.36, 32.6453) (-32.7077, 32.7668) (-32.3876, 32.7668) knots 0 0 0 1 2 2 2
  line L505 (-33.5342, 32.5966) -> (-33.36, 32.6453) construction
  line L506 (-33.36, 32.6453) -> (-32.7077, 32.7668) construction
  line L507 (-32.7077, 32.7668) -> (-32.3876, 32.7668) construction
  spline S84 degree 2 poles (-32.3876, 32.7668) (-31.9986, 32.7668) (-31.4678, 32.6453) (-31.2571, 32.4872) knots 0 0 0 1 2 2 2
  line L508 (-32.3876, 32.7668) -> (-31.9986, 32.7668) construction
  line L509 (-31.9986, 32.7668) -> (-31.4678, 32.6453) construction
  line L510 (-31.4678, 32.6453) -> (-31.2571, 32.4872) construction
  spline S85 degree 2 poles (-31.2571, 32.4872) (-31.0504, 32.3333) (-30.8479, 31.843) (-30.8479, 31.4905) knots 0 0 0 1 2 2 2
  line L511 (-31.2571, 32.4872) -> (-31.0504, 32.3333) construction
  line L512 (-31.0504, 32.3333) -> (-30.8479, 31.843) construction
  line L513 (-30.8479, 31.843) -> (-30.8479, 31.4905) construction
  spline S86 degree 2 poles (-31.4799, 29.3227) (-31.5569, 29.266) (-31.8162, 29.0634) (-31.9378, 29.0026) knots 0 0 0 1 2 2 2
  line L514 (-31.4799, 29.3227) -> (-31.5569, 29.266) construction
  line L515 (-31.5569, 29.266) -> (-31.8162, 29.0634) construction
  line L516 (-31.8162, 29.0634) -> (-31.9378, 29.0026) construction
  spline S87 degree 2 poles (-28.3965, 28.8527) (-28.6761, 28.8527) (-29.1055, 28.9824) (-29.3284, 29.1161) knots 0 0 0 1 2 2 2
  line L517 (-28.3965, 28.8527) -> (-28.6761, 28.8527) construction
  line L518 (-28.6761, 28.8527) -> (-29.1055, 28.9824) construction
  line L519 (-29.1055, 28.9824) -> (-29.3284, 29.1161) construction
  spline S88 degree 2 poles (-29.3284, 32.2846) (-29.0934, 32.4994) (-28.518, 32.783) (-28.1817, 32.783) knots 0 0 0 1 2 2 2
  line L520 (-29.3284, 32.2846) -> (-29.0934, 32.4994) construction
  line L521 (-29.0934, 32.4994) -> (-28.518, 32.783) construction
  line L522 (-28.518, 32.783) -> (-28.1817, 32.783) construction
  spline S89 degree 2 poles (-28.1817, 32.783) (-27.5375, 32.783) (-26.8162, 31.7619) (-26.8162, 30.903) knots 0 0 0 1 2 2 2
  line L523 (-28.1817, 32.783) -> (-27.5375, 32.783) construction
  line L524 (-27.5375, 32.783) -> (-26.8162, 31.7619) construction
  line L525 (-26.8162, 31.7619) -> (-26.8162, 30.903) construction
  spline S90 degree 2 poles (-26.8162, 30.903) (-26.8162, 29.9629) (-27.7117, 28.8527) (-28.3965, 28.8527) knots 0 0 0 1 2 2 2
  line L526 (-26.8162, 30.903) -> (-26.8162, 29.9629) construction
  line L527 (-26.8162, 29.9629) -> (-27.7117, 28.8527) construction
  line L528 (-27.7117, 28.8527) -> (-28.3965, 28.8527) construction
  spline S91 degree 2 poles (-25.3414, 30.4694) (-25.8114, 30.6072) (-26.2449, 31.1501) (-26.2449, 31.608) knots 0 0 0 1 2 2 2
  line L529 (-25.3414, 30.4694) -> (-25.8114, 30.6072) construction
  line L530 (-25.8114, 30.6072) -> (-26.2449, 31.1501) construction
  line L531 (-26.2449, 31.1501) -> (-26.2449, 31.608) construction
  spline S92 degree 2 poles (-26.2449, 31.608) (-26.2449, 31.8876) (-25.9978, 32.3089) (-25.7911, 32.4508) knots 0 0 0 1 2 2 2
  line L532 (-26.2449, 31.608) -> (-26.2449, 31.8876) construction
  line L533 (-26.2449, 31.8876) -> (-25.9978, 32.3089) construction
  line L534 (-25.9978, 32.3089) -> (-25.7911, 32.4508) construction
  spline S93 degree 2 poles (-25.7911, 32.4508) (-25.625, 32.5683) (-25.1104, 32.6777) (-24.7944, 32.6777) knots 0 0 0 1 2 2 2
  line L535 (-25.7911, 32.4508) -> (-25.625, 32.5683) construction
  line L536 (-25.625, 32.5683) -> (-25.1104, 32.6777) construction
  line L537 (-25.1104, 32.6777) -> (-24.7944, 32.6777) construction
  spline S94 degree 2 poles (-22.7117, 29.4645) (-22.3916, 29.9872) (-21.9864, 31.6769) (-21.9864, 32.6777) knots 0 0 0 1 2 2 2
  line L538 (-22.7117, 29.4645) -> (-22.3916, 29.9872) construction
  line L539 (-22.3916, 29.9872) -> (-21.9864, 31.6769) construction
  line L540 (-21.9864, 31.6769) -> (-21.9864, 32.6777) construction
  spline S95 degree 2 poles (-31.877, 23.4404) (-31.484, 23.4526) (-31.0221, 23.8213) (-30.8803, 24.1698) knots 0 0 0 1 2 2 2
  line L541 (-31.877, 23.4404) -> (-31.484, 23.4526) construction
  line L542 (-31.484, 23.4526) -> (-31.0221, 23.8213) construction
  line L543 (-31.0221, 23.8213) -> (-30.8803, 24.1698) construction
  spline S96 degree 2 poles (-30.8803, 24.1698) (-30.8195, 24.3197) (-30.7222, 24.5912) (-30.6939, 24.6884) knots 0 0 0 1 2 2 2
  line L544 (-30.8803, 24.1698) -> (-30.8195, 24.3197) construction
  line L545 (-30.8195, 24.3197) -> (-30.7222, 24.5912) construction
  line L546 (-30.7222, 24.5912) -> (-30.6939, 24.6884) construction
  spline S97 degree 2 poles (-30.6939, 24.6884) (-30.4913, 25.2597) (-29.8673, 25.6933) (-29.3122, 25.6933) knots 0 0 0 1 2 2 2
  line L547 (-30.6939, 24.6884) -> (-30.4913, 25.2597) construction
  line L548 (-30.4913, 25.2597) -> (-29.8673, 25.6933) construction
  line L549 (-29.8673, 25.6933) -> (-29.3122, 25.6933) construction
  spline S98 degree 2 poles (-29.2717, 25.1017) (-29.685, 25.1017) (-30.0132, 24.7816) (-30.1509, 24.3359) knots 0 0 0 1 2 2 2
  line L550 (-29.2717, 25.1017) -> (-29.685, 25.1017) construction
  line L551 (-29.685, 25.1017) -> (-30.0132, 24.7816) construction
  line L552 (-30.0132, 24.7816) -> (-30.1509, 24.3359) construction
  spline S99 degree 2 poles (-30.1509, 24.3359) (-30.2887, 23.8942) (-30.6291, 23.481) (-30.8722, 23.3229) knots 0 0 0 1 2 2 2
  line L553 (-30.1509, 24.3359) -> (-30.2887, 23.8942) construction
  line L554 (-30.2887, 23.8942) -> (-30.6291, 23.481) construction
  line L555 (-30.6291, 23.481) -> (-30.8722, 23.3229) construction
  spline S100 degree 2 poles (22.2959, 29.4639) (22.069, 29.2857) (21.5666, 29.1601) (21.2181, 29.1601) knots 0 0 0 1 2 2 2
  line L556 (22.2959, 29.4639) -> (22.069, 29.2857) construction
  line L557 (22.069, 29.2857) -> (21.5666, 29.1601) construction
  line L558 (21.5666, 29.1601) -> (21.2181, 29.1601) construction
  spline S101 degree 2 poles (21.1209, 32.9121) (21.5342, 32.9121) (21.915, 32.8635) (22.1055, 32.7581) knots 0 0 0 1 2 2 2
  line L559 (21.1209, 32.9121) -> (21.5342, 32.9121) construction
  line L560 (21.5342, 32.9121) -> (21.915, 32.8635) construction
  line L561 (21.915, 32.8635) -> (22.1055, 32.7581) construction
  spline S102 degree 2 poles (22.1055, 32.7581) (22.304, 32.6487) (22.4904, 32.2921) (22.4904, 32.049) knots 0 0 0 1 2 2 2
  line L562 (22.1055, 32.7581) -> (22.304, 32.6487) construction
  line L563 (22.304, 32.6487) -> (22.4904, 32.2921) construction
  line L564 (22.4904, 32.2921) -> (22.4904, 32.049) construction
  spline S103 degree 2 poles (22.4904, 32.049) (22.4904, 31.7816) (22.1946, 31.3521) (21.9515, 31.2346) knots 0 0 0 1 2 2 2
  line L565 (22.4904, 32.049) -> (22.4904, 31.7816) construction
  line L566 (22.4904, 31.7816) -> (22.1946, 31.3521) construction
  line L567 (22.1946, 31.3521) -> (21.9515, 31.2346) construction
  line L568 (21.9515, 31.2346) -> (21.9677, 31.2143)
  spline S104 degree 2 poles (21.9677, 31.2143) (22.2716, 31.1333) (22.6849, 30.6633) (22.6849, 30.2946) knots 0 0 0 1 2 2 2
  line L569 (21.9677, 31.2143) -> (22.2716, 31.1333) construction
  line L570 (22.2716, 31.1333) -> (22.6849, 30.6633) construction
  line L571 (22.6849, 30.6633) -> (22.6849, 30.2946) construction
  spline S105 degree 2 poles (22.6849, 30.2946) (22.6849, 30.0231) (22.4783, 29.6017) (22.2959, 29.4639) knots 0 0 0 1 2 2 2
  line L572 (22.6849, 30.2946) -> (22.6849, 30.0231) construction
  line L573 (22.6849, 30.0231) -> (22.4783, 29.6017) construction
  line L574 (22.4783, 29.6017) -> (22.2959, 29.4639) construction
  spline S106 degree 2 poles (32.5552, 29.468) (32.3324, 29.3019) (31.83, 29.1601) (31.4369, 29.1601) knots 0 0 0 1 2 2 2
  line L575 (32.5552, 29.468) -> (32.3324, 29.3019) construction
  line L576 (32.3324, 29.3019) -> (31.83, 29.1601) construction
  line L577 (31.83, 29.1601) -> (31.4369, 29.1601) construction
  spline S107 degree 2 poles (31.4531, 31.4494) (31.8745, 31.4494) (32.3405, 31.3602) (32.5714, 31.19) knots 0 0 0 1 2 2 2
  line L578 (31.4531, 31.4494) -> (31.8745, 31.4494) construction
  line L579 (31.8745, 31.4494) -> (32.3405, 31.3602) construction